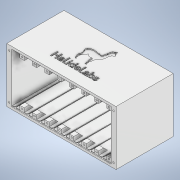
# Autodesk Inventor part: obudowa_główna
Saved by Autodesk Inventor 2020 (Build 240168000, 168)
## iProperties
Created: 2020-04-06
Part Number: obudowa_główna
Material: Tworzywo sztuczne ABS
Document SubType Name: Modeling
Designer: Bartek
Density: 1.06 g/cm^3
Appearance: Gładki — biały
Mass: 835.095 g
Surface Area: 2333.52 cm^2
Volume: 787.826 cm^3
Author: Bartek
Autodesk Inventor part; units mm, degrees
(part 1 of 3)
sketch "Szkic1" plane through (0, 0, 0) normal (0, 0, 1) x (1, 0, 0)
  line L0 (-110, 55) -> (110, 55)
  line L1 (110, 55) -> (110, -55)
  line L2 (110, -55) -> (-110, -55)
  line L3 (-110, -55) -> (-110, 55)
  line L4 (-110, 55) -> (110, -55) construction
  line L5 (110, 55) -> (-110, -55) construction
  point P0 (0, 0)
  dimension "d0" = 220
  dimension "d1" = 110
  constraints: 12 end point, 2 midpoint, 2 parallel, 1 horizontal, 1 perpendicular
  measures "d0" distance of L1.end L2.end
  measures "d1" distance of L0.end L1.end
extrude "Wyciągnięcie proste1" add sketch "Szkic1" along normal blind 115.25
sketch "Szkic2" plane through (0, 0, 115.25) normal (0, 0, 1) x (1, 0, 0)
  line L0 (-110, 55) -> (-110, -55) projected
  line L1 (-95, 50.2) -> (-93.2, 50.2)
  line L2 (-93.2, 50.2) -> (-93.2, 49)
  line L3 (-93.2, 49) -> (-95, 49)
  line L4 (-95, 49) -> (-95, 50.2)
  line L5 (-95, 50.2) -> (-93.2, 49) construction
  line L6 (-93.2, 50.2) -> (-95, 49) construction
  line L7 (110, 55) -> (-110, 55) projected
  line L8 (-70, 49) -> (-70, 50.2)
  line L9 (-68.2, 49) -> (-70, 49)
  line L10 (-68.2, 50.2) -> (-68.2, 49)
  line L11 (-70, 50.2) -> (-68.2, 50.2)
  line L12 (-45, 49) -> (-45, 50.2)
  line L13 (-43.2, 49) -> (-45, 49)
  line L14 (-43.2, 50.2) -> (-43.2, 49)
  line L15 (-45, 50.2) -> (-43.2, 50.2)
  line L16 (-20, 49) -> (-20, 50.2)
  line L17 (-18.2, 49) -> (-20, 49)
  line L18 (-18.2, 50.2) -> (-18.2, 49)
  line L19 (-20, 50.2) -> (-18.2, 50.2)
  line L20 (5, 49) -> (5, 50.2)
  line L21 (6.8, 49) -> (5, 49)
  line L22 (6.8, 50.2) -> (6.8, 49)
  line L23 (5, 50.2) -> (6.8, 50.2)
  line L24 (30, 49) -> (30, 50.2)
  line L25 (31.8, 49) -> (30, 49)
  line L26 (31.8, 50.2) -> (31.8, 49)
  line L27 (30, 50.2) -> (31.8, 50.2)
  line L28 (55, 49) -> (55, 50.2)
  line L29 (56.8, 49) -> (55, 49)
  line L30 (56.8, 50.2) -> (56.8, 49)
  line L31 (55, 50.2) -> (56.8, 50.2)
  line L32 (80, 49) -> (80, 50.2)
  line L33 (81.8, 49) -> (80, 49)
  line L34 (81.8, 50.2) -> (81.8, 49)
  line L35 (80, 50.2) -> (81.8, 50.2)
  line L36 (-110, 0) -> (110, 0)
  line L37 (-95, -50.2) -> (-93.2, -50.2)
  line L38 (-93.2, -50.2) -> (-93.2, -49)
  line L39 (-93.2, -49) -> (-95, -49)
  line L40 (-95, -49) -> (-95, -50.2)
  line L41 (-95, -50.2) -> (-93.2, -49) construction
  line L42 (-93.2, -50.2) -> (-95, -49) construction
  line L43 (-70, -49) -> (-70, -50.2)
  line L44 (-68.2, -49) -> (-70, -49)
  line L45 (-68.2, -50.2) -> (-68.2, -49)
  line L46 (-70, -50.2) -> (-68.2, -50.2)
  line L47 (-45, -49) -> (-45, -50.2)
  line L48 (-43.2, -49) -> (-45, -49)
  line L49 (-43.2, -50.2) -> (-43.2, -49)
  line L50 (-45, -50.2) -> (-43.2, -50.2)
  line L51 (-20, -49) -> (-20, -50.2)
  line L52 (-18.2, -49) -> (-20, -49)
  line L53 (-18.2, -50.2) -> (-18.2, -49)
  line L54 (-20, -50.2) -> (-18.2, -50.2)
  line L55 (5, -49) -> (5, -50.2)
  line L56 (6.8, -49) -> (5, -49)
  line L57 (6.8, -50.2) -> (6.8, -49)
  line L58 (5, -50.2) -> (6.8, -50.2)
  line L59 (30, -49) -> (30, -50.2)
  line L60 (31.8, -49) -> (30, -49)
  line L61 (31.8, -50.2) -> (31.8, -49)
  line L62 (30, -50.2) -> (31.8, -50.2)
  line L63 (55, -49) -> (55, -50.2)
  line L64 (56.8, -49) -> (55, -49)
  line L65 (56.8, -50.2) -> (56.8, -49)
  line L66 (55, -50.2) -> (56.8, -50.2)
  line L67 (80, -49) -> (80, -50.2)
  line L68 (81.8, -49) -> (80, -49)
  line L69 (81.8, -50.2) -> (81.8, -49)
  line L70 (80, -50.2) -> (81.8, -50.2)
  line L71 (-110, -55) -> (110, -55) projected
  point P0 (0, 0)
  point P1 (-94.1, 49.6)
  point P2 (-94.1, -49.6)
  dimension "d7" = 1.8
  dimension "d11" = 15
  dimension "d12" = 4.8
  dimension "d13" = 1.2
  dimension "d17" = 25
  dimension "d56" = 4.8
  dimension "d129" = 1.2
  constraints: 138 end point, 33 symmetric about line, 5 midpoint, 3 horizontal, 2 parallel, 1 collinear, 1 perpendicular, 55 other
  measures "d7" distance between parallel lines of L2 L4
  measures "d11" horizontal distance of L0.start L1.start
  measures "d12" distance between parallel lines of L7 L1
  measures "d13" distance between parallel lines of L1 L3
  measures "d17" distance of L3.end L8.start
  measures "d56" distance from line of L71 L37.start
  measures "d129" distance between parallel lines of L39 L37
extrude "Wyciągnięcie proste2" cut sketch "Szkic2" against normal blind 103.65
sketch "Szkic3" plane through (0, 0, 115.25) normal (0, 0, 1) x (1, 0, 0)
  line L0 (-95, 49) -> (-100, 49)
  line L1 (-100, 49) -> (-100, -49)
  line L2 (-100, -49) -> (100, -49)
  line L3 (100, -49) -> (100, 49)
  line L4 (100, 49) -> (-100, 49)
  line L5 (110, -55) -> (110, 55) projected
  line L6 (-110, 55) -> (-110, -55) projected
  line L7 (110, 55) -> (-110, 55) projected
  point P0 (0, 0)
  dimension "d24" = 5
  dimension "d25" = 98
  dimension "d26" = 200
  dimension "d27" = 98
  dimension "d28" = 90
  dimension "d29" = 10
  dimension "d30" = 10
  dimension "d31" = 6
  dimension "d63" = 6
  constraints: 10 end point, 3 perpendicular, 1 horizontal
  measures "d24" distance of L0.start L0.end
  measures "d25" distance of L0.end L1.end
  measures "d26" distance of L1.end L2.end
  measures "d27" distance of L2.end L3.end
  measures "d28" angle of L3 L2
  measures "d29" distance between parallel lines of L5 L3
  measures "d30" distance between parallel lines of L1 L6
  measures "d31" distance from line of L5.start L2
  measures "d63" distance from line of L7 L0.start
extrude "Wyciągnięcie proste3" cut sketch "Szkic3" against normal blind 106.61
ref_plane "Płaszczyzna konstrukcyjna2" through (0, 0, 115.25) normal (0, 0, 1) x (1, 0, 0)
sketch "Szkic4" plane through (0, 0, 115.25) normal (0, 0, 1) x (1, 0, 0)
  line L0 (-94.1, 52.3714) -> (-94.1, 48.8259)
  line L1 (-93.2, 50.2) -> (-93.2, 49) projected
  line L2 (-95, 49) -> (-95, 50.2) projected
  line L3 (-100, 0) -> (99.7125, 0)
  line L4 (-95, 50.2) -> (-93.2, 50.2) projected
  circle A0 centre (-80.7, 45.2) radius 1.5
  line L5 (-85.1, 49.2) -> (-85.1, 41.2)
  line L6 (-85.1, 41.2) -> (-76.3, 41.2)
  line L7 (-76.3, 41.2) -> (-76.3, 49.2)
  line L8 (-76.3, 49.2) -> (-85.1, 49.2)
  line L9 (-80.6711, 45.15) -> (-80.7289, 45.15)
  line L10 (-80.7289, 45.15) -> (-80.7577, 45.2)
  line L11 (-80.7577, 45.2) -> (-80.7289, 45.25)
  line L12 (-80.7289, 45.25) -> (-80.6711, 45.25)
  line L13 (-80.6711, 45.25) -> (-80.6423, 45.2)
  line L14 (-80.6423, 45.2) -> (-80.6711, 45.15)
  line L15 (-60.1, 49.2) -> (-60.1, 41.2)
  line L16 (-60.1, 41.2) -> (-51.3, 41.2)
  line L17 (-51.3, 49.2) -> (-60.1, 49.2)
  line L18 (-51.3, 41.2) -> (-51.3, 49.2)
  line L19 (-55.6711, 45.25) -> (-55.6423, 45.2)
  line L20 (-55.7289, 45.25) -> (-55.6711, 45.25)
  line L21 (-55.7577, 45.2) -> (-55.7289, 45.25)
  line L22 (-55.7289, 45.15) -> (-55.7577, 45.2)
  line L23 (-55.6711, 45.15) -> (-55.7289, 45.15)
  line L24 (-55.6423, 45.2) -> (-55.6711, 45.15)
  circle A1 centre (-55.7, 45.2) radius 1.5
  line L25 (-35.1, 49.2) -> (-35.1, 41.2)
  line L26 (-35.1, 41.2) -> (-26.3, 41.2)
  line L27 (-26.3, 49.2) -> (-35.1, 49.2)
  line L28 (-26.3, 41.2) -> (-26.3, 49.2)
  line L29 (-30.6711, 45.25) -> (-30.6423, 45.2)
  line L30 (-30.7289, 45.25) -> (-30.6711, 45.25)
  line L31 (-30.7577, 45.2) -> (-30.7289, 45.25)
  line L32 (-30.7289, 45.15) -> (-30.7577, 45.2)
  line L33 (-30.6711, 45.15) -> (-30.7289, 45.15)
  line L34 (-30.6423, 45.2) -> (-30.6711, 45.15)
  circle A2 centre (-30.7, 45.2) radius 1.5
  line L35 (-10.1, 49.2) -> (-10.1, 41.2)
  line L36 (-10.1, 41.2) -> (-1.3, 41.2)
  line L37 (-1.3, 49.2) -> (-10.1, 49.2)
  line L38 (-1.3, 41.2) -> (-1.3, 49.2)
  line L39 (-5.6711, 45.25) -> (-5.6423, 45.2)
  line L40 (-5.7289, 45.25) -> (-5.6711, 45.25)
  line L41 (-5.7577, 45.2) -> (-5.7289, 45.25)
  line L42 (-5.7289, 45.15) -> (-5.7577, 45.2)
  line L43 (-5.6711, 45.15) -> (-5.7289, 45.15)
  line L44 (-5.6423, 45.2) -> (-5.6711, 45.15)
  circle A3 centre (-5.7, 45.2) radius 1.5
  line L45 (14.9, 49.2) -> (14.9, 41.2)
  line L46 (14.9, 41.2) -> (23.7, 41.2)
  line L47 (23.7, 49.2) -> (14.9, 49.2)
  line L48 (23.7, 41.2) -> (23.7, 49.2)
  line L49 (19.3289, 45.25) -> (19.3577, 45.2)
  line L50 (19.2711, 45.25) -> (19.3289, 45.25)
  line L51 (19.2423, 45.2) -> (19.2711, 45.25)
  line L52 (19.2711, 45.15) -> (19.2423, 45.2)
  line L53 (19.3289, 45.15) -> (19.2711, 45.15)
  line L54 (19.3577, 45.2) -> (19.3289, 45.15)
  circle A4 centre (19.3, 45.2) radius 1.5
  line L55 (39.9, 49.2) -> (39.9, 41.2)
  line L56 (39.9, 41.2) -> (48.7, 41.2)
  line L57 (48.7, 49.2) -> (39.9, 49.2)
  line L58 (48.7, 41.2) -> (48.7, 49.2)
  line L59 (44.3289, 45.25) -> (44.3577, 45.2)
  line L60 (44.2711, 45.25) -> (44.3289, 45.25)
  line L61 (44.2423, 45.2) -> (44.2711, 45.25)
  line L62 (44.2711, 45.15) -> (44.2423, 45.2)
  line L63 (44.3289, 45.15) -> (44.2711, 45.15)
  line L64 (44.3577, 45.2) -> (44.3289, 45.15)
  circle A5 centre (44.3, 45.2) radius 1.5
  line L65 (64.9, 49.2) -> (64.9, 41.2)
  line L66 (64.9, 41.2) -> (73.7, 41.2)
  line L67 (73.7, 49.2) -> (64.9, 49.2)
  line L68 (73.7, 41.2) -> (73.7, 49.2)
  line L69 (69.3289, 45.25) -> (69.3577, 45.2)
  line L70 (69.2711, 45.25) -> (69.3289, 45.25)
  line L71 (69.2423, 45.2) -> (69.2711, 45.25)
  line L72 (69.2711, 45.15) -> (69.2423, 45.2)
  line L73 (69.3289, 45.15) -> (69.2711, 45.15)
  line L74 (69.3577, 45.2) -> (69.3289, 45.15)
  circle A6 centre (69.3, 45.2) radius 1.5
  line L75 (89.9, 49.2) -> (89.9, 41.2)
  line L76 (89.9, 41.2) -> (98.7, 41.2)
  line L77 (98.7, 49.2) -> (89.9, 49.2)
  line L78 (98.7, 41.2) -> (98.7, 49.2)
  line L79 (94.3289, 45.25) -> (94.3577, 45.2)
  line L80 (94.2711, 45.25) -> (94.3289, 45.25)
  line L81 (94.2423, 45.2) -> (94.2711, 45.25)
  line L82 (94.2711, 45.15) -> (94.2423, 45.2)
  line L83 (94.3289, 45.15) -> (94.2711, 45.15)
  line L84 (94.3577, 45.2) -> (94.3289, 45.15)
  circle A7 centre (94.3, 45.2) radius 1.5
  line L85 (-94.1, -52.3714) -> (-94.1, -48.8259)
  line L86 (-93.2, -50.2) -> (-93.2, -49)
  line L87 (-95, -49) -> (-95, -50.2)
  line L88 (-95, -50.2) -> (-93.2, -50.2)
  circle A8 centre (-80.7, -45.2) radius 1.5
  line L89 (-85.1, -49.2) -> (-85.1, -41.2)
  line L90 (-85.1, -41.2) -> (-76.3, -41.2)
  line L91 (-76.3, -41.2) -> (-76.3, -49.2)
  line L92 (-76.3, -49.2) -> (-85.1, -49.2)
  line L93 (-80.6711, -45.15) -> (-80.7289, -45.15)
  line L94 (-80.7289, -45.15) -> (-80.7577, -45.2)
  line L95 (-80.7577, -45.2) -> (-80.7289, -45.25)
  line L96 (-80.7289, -45.25) -> (-80.6711, -45.25)
  line L97 (-80.6711, -45.25) -> (-80.6423, -45.2)
  line L98 (-80.6423, -45.2) -> (-80.6711, -45.15)
  line L99 (-60.1, -49.2) -> (-60.1, -41.2)
  line L100 (-60.1, -41.2) -> (-51.3, -41.2)
  line L101 (-51.3, -49.2) -> (-60.1, -49.2)
  line L102 (-51.3, -41.2) -> (-51.3, -49.2)
  line L103 (-55.6711, -45.25) -> (-55.6423, -45.2)
  line L104 (-55.7289, -45.25) -> (-55.6711, -45.25)
  line L105 (-55.7577, -45.2) -> (-55.7289, -45.25)
  line L106 (-55.7289, -45.15) -> (-55.7577, -45.2)
  line L107 (-55.6711, -45.15) -> (-55.7289, -45.15)
  line L108 (-55.6423, -45.2) -> (-55.6711, -45.15)
  circle A9 centre (-55.7, -45.2) radius 1.5
  line L109 (-35.1, -49.2) -> (-35.1, -41.2)
  line L110 (-35.1, -41.2) -> (-26.3, -41.2)
  line L111 (-26.3, -49.2) -> (-35.1, -49.2)
  line L112 (-26.3, -41.2) -> (-26.3, -49.2)
  line L113 (-30.6711, -45.25) -> (-30.6423, -45.2)
  line L114 (-30.7289, -45.25) -> (-30.6711, -45.25)
  line L115 (-30.7577, -45.2) -> (-30.7289, -45.25)
  line L116 (-30.7289, -45.15) -> (-30.7577, -45.2)
  line L117 (-30.6711, -45.15) -> (-30.7289, -45.15)
  line L118 (-30.6423, -45.2) -> (-30.6711, -45.15)
  circle A10 centre (-30.7, -45.2) radius 1.5
  line L119 (-10.1, -49.2) -> (-10.1, -41.2)
  line L120 (-10.1, -41.2) -> (-1.3, -41.2)
  line L121 (-1.3, -49.2) -> (-10.1, -49.2)
  line L122 (-1.3, -41.2) -> (-1.3, -49.2)
  line L123 (-5.6711, -45.25) -> (-5.6423, -45.2)
  line L124 (-5.7289, -45.25) -> (-5.6711, -45.25)
  line L125 (-5.7577, -45.2) -> (-5.7289, -45.25)
  line L126 (-5.7289, -45.15) -> (-5.7577, -45.2)
  line L127 (-5.6711, -45.15) -> (-5.7289, -45.15)
  line L128 (-5.6423, -45.2) -> (-5.6711, -45.15)
  circle A11 centre (-5.7, -45.2) radius 1.5
  line L129 (14.9, -49.2) -> (14.9, -41.2)
  line L130 (14.9, -41.2) -> (23.7, -41.2)
  line L131 (23.7, -49.2) -> (14.9, -49.2)
  line L132 (23.7, -41.2) -> (23.7, -49.2)
  line L133 (19.3289, -45.25) -> (19.3577, -45.2)
  line L134 (19.2711, -45.25) -> (19.3289, -45.25)
  line L135 (19.2423, -45.2) -> (19.2711, -45.25)
  line L136 (19.2711, -45.15) -> (19.2423, -45.2)
  line L137 (19.3289, -45.15) -> (19.2711, -45.15)
  line L138 (19.3577, -45.2) -> (19.3289, -45.15)
  circle A12 centre (19.3, -45.2) radius 1.5
  line L139 (39.9, -49.2) -> (39.9, -41.2)
  line L140 (39.9, -41.2) -> (48.7, -41.2)
  line L141 (48.7, -49.2) -> (39.9, -49.2)
  line L142 (48.7, -41.2) -> (48.7, -49.2)
  line L143 (44.3289, -45.25) -> (44.3577, -45.2)
  line L144 (44.2711, -45.25) -> (44.3289, -45.25)
  line L145 (44.2423, -45.2) -> (44.2711, -45.25)
  line L146 (44.2711, -45.15) -> (44.2423, -45.2)
  line L147 (44.3289, -45.15) -> (44.2711, -45.15)
  line L148 (44.3577, -45.2) -> (44.3289, -45.15)
  circle A13 centre (44.3, -45.2) radius 1.5
  line L149 (64.9, -49.2) -> (64.9, -41.2)
  line L150 (64.9, -41.2) -> (73.7, -41.2)
  line L151 (73.7, -49.2) -> (64.9, -49.2)
  line L152 (73.7, -41.2) -> (73.7, -49.2)
  line L153 (69.3289, -45.25) -> (69.3577, -45.2)
  line L154 (69.2711, -45.25) -> (69.3289, -45.25)
  line L155 (69.2423, -45.2) -> (69.2711, -45.25)
  line L156 (69.2711, -45.15) -> (69.2423, -45.2)
  line L157 (69.3289, -45.15) -> (69.2711, -45.15)
  line L158 (69.3577, -45.2) -> (69.3289, -45.15)
  circle A14 centre (69.3, -45.2) radius 1.5
  line L159 (89.9, -49.2) -> (89.9, -41.2)
  line L160 (89.9, -41.2) -> (98.7, -41.2)
  line L161 (98.7, -49.2) -> (89.9, -49.2)
  line L162 (98.7, -41.2) -> (98.7, -49.2)
  line L163 (94.3289, -45.25) -> (94.3577, -45.2)
  line L164 (94.2711, -45.25) -> (94.3289, -45.25)
  line L165 (94.2423, -45.2) -> (94.2711, -45.25)
  line L166 (94.2711, -45.15) -> (94.2423, -45.2)
  line L167 (94.3289, -45.15) -> (94.2711, -45.15)
  line L168 (94.3577, -45.2) -> (94.3289, -45.15)
  circle A15 centre (94.3, -45.2) radius 1.5
  point P0 (0, 0)
  dimension "d35" = 1.8
  dimension "d36" = 0.9
  dimension "d39" = 3
  dimension "d40" = 5
  dimension "d41" = 13.4
  dimension "d42" = 8
  dimension "d43" = 8.8
  dimension "d44" = 4.4
  dimension "d45" = 14.3
  dimension "d46" = 0.1
  dimension "d49" = 25
  dimension "d64" = 4
  constraints: 332 end point, 95 symmetric about line, 16 centre point, 3 vertical, 2 coincident, 2 horizontal, 2 perpendicular, 1 collinear, 1 parallel, 173 other
  measures "d35" distance between parallel lines of L1 L2
  measures "d36" distance between parallel lines of L0 L2
  measures "d39" diameter of A0
  measures "d40" distance from line of L4 A0.centre
  measures "d41" distance from line of A0.centre L0
  measures "d42" distance of L5.start L5.end
  measures "d43" distance of L5.end L6.end
  measures "d44" distance from line of L5 A0.centre
  measures "d45" distance from line of L2 A0.centre
  measures "d46" vertical distance of L12.end L9.end
  measures "d49" distance of L5.start L15.start
  measures "d64" distance from line of L6 A0.centre
extrude "Wyciągnięcie proste4" add sketch "Szkic4" against normal blind 106.61 contours L8 L7 L6 L5 | L17 L18 L16 L15 | L27 L28 L26 L25 | L37 L38 L36 L35 | L47 L48 L46 L45 | L57 L58 L56 L55 | L67 L68 L66 L65 | L77 L78 L76 L75 | L89 L90 L91 L92 | L99 L100 L102 L101 | L109 L110 L112 L111 | L119 L120 L122 L121 | L129 L130 L132 L131 | L139 L140 L142 L141 | L149 L150 L152 L151 | L159 L160 L162 L161
sketch "Szkic5" plane through (0, 0, 115.25) normal (0, 0, 1) x (1, 0, 0)
  line L0 (100, 49) -> (100, -49) projected
  line L1 (-100, -49) -> (-100, 49) projected
  line L2 (-100, 50.2) -> (100, 50.2)
  line L3 (100, 50.2) -> (100, -50.2)
  line L4 (100, -50.2) -> (-100, -50.2)
  line L5 (-100, -50.2) -> (-100, 50.2)
  line L6 (-100, 50.2) -> (100, -50.2) construction
  line L7 (100, 50.2) -> (-100, -50.2) construction
  point P0 (0, 0)
  point P1 (100, -49)
  point P2 (-100, 49)
  point P3 (-100, -49)
  dimension "d57" = 200
  dimension "d58" = 98
  dimension "d59" = 200
  dimension "d60" = 100.4
  constraints: 12 end point, 2 midpoint, 2 parallel, 1 horizontal, 1 perpendicular
  measures "d57" distance between parallel lines of L0 L1
  measures "d58" distance of L1.end L1.start
  measures "d59" distance between parallel lines of L3 L5
  measures "d60" distance between parallel lines of L2 L4
extrude "Wyciągnięcie proste5" cut sketch "Szkic5" against normal blind 1.6
ref_plane "Płaszczyzna konstrukcyjna5" through (-51.3, -49, 10) normal (0, 1, 0) x (1, 0, 0)
sketch "Szkic7" plane through (-51.3, -49, 10) normal (0, 1, 0) x (1, 0, 0)
  line L0 (-44.5014, -102.9088) -> (-43.7341, -100.0451)
  line L1 (-44.8189, -104.0803) -> (-39.2569, -104.0803) construction
  line L2 (-42.8, -98.9304) -> (-42.8, -103.8241)
  line L3 (-41.9, -103.65) -> (-41.9, -1.6) projected
  arc A0 (-43.7341, -100.0451) -> (-43.7, -99.7863) centre (-44.7, -99.7863) ccw
  line L4 (-43.7, -103.65) -> (-43.7, -99.7863)
  line L5 (-43.7, -103.65) -> (-43.7, -1.6) projected
  arc A1 (-45.4673, -103.65) -> (-44.5014, -102.9088) centre (-45.4673, -102.65) ccw
  line L6 (-43.7, -103.65) -> (-45.4673, -103.65)
  line L7 (-41.0986, -102.9088) -> (-41.8659, -100.0451)
  arc A2 (-41.9, -99.7863) -> (-41.8659, -100.0451) centre (-40.9, -99.7863) ccw
  line L8 (-41.9, -103.65) -> (-41.9, -99.7863)
  arc A3 (-41.0986, -102.9088) -> (-40.1327, -103.65) centre (-40.1327, -102.65) ccw
  line L9 (-41.9, -103.65) -> (-40.1327, -103.65)
  line L10 (-19.5014, -102.9088) -> (-18.7341, -100.0451)
  arc A4 (-20.4673, -103.65) -> (-19.5014, -102.9088) centre (-20.4673, -102.65) ccw
  line L11 (-18.7, -103.65) -> (-18.7, -99.7863)
  arc A5 (-18.7341, -100.0451) -> (-18.7, -99.7863) centre (-19.7, -99.7863) ccw
  line L12 (-18.7, -103.65) -> (-20.4673, -103.65)
  arc A6 (-16.9, -99.7863) -> (-16.8659, -100.0451) centre (-15.9, -99.7863) ccw
  line L13 (-16.9, -103.65) -> (-16.9, -99.7863)
  line L14 (-16.0986, -102.9088) -> (-16.8659, -100.0451)
  arc A7 (-16.0986, -102.9088) -> (-15.1327, -103.65) centre (-15.1327, -102.65) ccw
  line L15 (-16.9, -103.65) -> (-15.1327, -103.65)
  line L16 (5.4986, -102.9088) -> (6.2659, -100.0451)
  arc A8 (4.5327, -103.65) -> (5.4986, -102.9088) centre (4.5327, -102.65) ccw
  line L17 (6.3, -103.65) -> (6.3, -99.7863)
  arc A9 (6.2659, -100.0451) -> (6.3, -99.7863) centre (5.3, -99.7863) ccw
  line L18 (6.3, -103.65) -> (4.5327, -103.65)
  arc A10 (8.1, -99.7863) -> (8.1341, -100.0451) centre (9.1, -99.7863) ccw
  line L19 (8.1, -103.65) -> (8.1, -99.7863)
  line L20 (8.9014, -102.9088) -> (8.1341, -100.0451)
  arc A11 (8.9014, -102.9088) -> (9.8673, -103.65) centre (9.8673, -102.65) ccw
  line L21 (8.1, -103.65) -> (9.8673, -103.65)
  line L22 (30.4986, -102.9088) -> (31.2659, -100.0451)
  arc A12 (29.5327, -103.65) -> (30.4986, -102.9088) centre (29.5327, -102.65) ccw
  line L23 (31.3, -103.65) -> (31.3, -99.7863)
  arc A13 (31.2659, -100.0451) -> (31.3, -99.7863) centre (30.3, -99.7863) ccw
  line L24 (31.3, -103.65) -> (29.5327, -103.65)
  arc A14 (33.1, -99.7863) -> (33.1341, -100.0451) centre (34.1, -99.7863) ccw
  line L25 (33.1, -103.65) -> (33.1, -99.7863)
  line L26 (33.9014, -102.9088) -> (33.1341, -100.0451)
  arc A15 (33.9014, -102.9088) -> (34.8673, -103.65) centre (34.8673, -102.65) ccw
  line L27 (33.1, -103.65) -> (34.8673, -103.65)
  line L28 (55.4986, -102.9088) -> (56.2659, -100.0451)
  arc A16 (54.5327, -103.65) -> (55.4986, -102.9088) centre (54.5327, -102.65) ccw
  line L29 (56.3, -103.65) -> (56.3, -99.7863)
  arc A17 (56.2659, -100.0451) -> (56.3, -99.7863) centre (55.3, -99.7863) ccw
  line L30 (56.3, -103.65) -> (54.5327, -103.65)
  arc A18 (58.1, -99.7863) -> (58.1341, -100.0451) centre (59.1, -99.7863) ccw
  line L31 (58.1, -103.65) -> (58.1, -99.7863)
  line L32 (58.9014, -102.9088) -> (58.1341, -100.0451)
  arc A19 (58.9014, -102.9088) -> (59.8673, -103.65) centre (59.8673, -102.65) ccw
  line L33 (58.1, -103.65) -> (59.8673, -103.65)
  line L34 (80.4986, -102.9088) -> (81.2659, -100.0451)
  arc A20 (79.5327, -103.65) -> (80.4986, -102.9088) centre (79.5327, -102.65) ccw
  line L35 (81.3, -103.65) -> (81.3, -99.7863)
  arc A21 (81.2659, -100.0451) -> (81.3, -99.7863) centre (80.3, -99.7863) ccw
  line L36 (81.3, -103.65) -> (79.5327, -103.65)
  arc A22 (83.1, -99.7863) -> (83.1341, -100.0451) centre (84.1, -99.7863) ccw
  line L37 (83.1, -103.65) -> (83.1, -99.7863)
  line L38 (83.9014, -102.9088) -> (83.1341, -100.0451)
  arc A23 (83.9014, -102.9088) -> (84.8673, -103.65) centre (84.8673, -102.65) ccw
  line L39 (83.1, -103.65) -> (84.8673, -103.65)
  line L40 (105.4986, -102.9088) -> (106.2659, -100.0451)
  arc A24 (104.5327, -103.65) -> (105.4986, -102.9088) centre (104.5327, -102.65) ccw
  line L41 (106.3, -103.65) -> (106.3, -99.7863)
  arc A25 (106.2659, -100.0451) -> (106.3, -99.7863) centre (105.3, -99.7863) ccw
  line L42 (106.3, -103.65) -> (104.5327, -103.65)
  arc A26 (108.1, -99.7863) -> (108.1341, -100.0451) centre (109.1, -99.7863) ccw
  line L43 (108.1, -103.65) -> (108.1, -99.7863)
  line L44 (108.9014, -102.9088) -> (108.1341, -100.0451)
  arc A27 (108.9014, -102.9088) -> (109.8673, -103.65) centre (109.8673, -102.65) ccw
  line L45 (108.1, -103.65) -> (109.8673, -103.65)
  line L46 (130.4986, -102.9088) -> (131.2659, -100.0451)
  arc A28 (129.5327, -103.65) -> (130.4986, -102.9088) centre (129.5327, -102.65) ccw
  line L47 (131.3, -103.65) -> (131.3, -99.7863)
  arc A29 (131.2659, -100.0451) -> (131.3, -99.7863) centre (130.3, -99.7863) ccw
  line L48 (131.3, -103.65) -> (129.5327, -103.65)
  arc A30 (133.1, -99.7863) -> (133.1341, -100.0451) centre (134.1, -99.7863) ccw
  line L49 (133.1, -103.65) -> (133.1, -99.7863)
  line L50 (133.9014, -102.9088) -> (133.1341, -100.0451)
  arc A31 (133.9014, -102.9088) -> (134.8673, -103.65) centre (134.8673, -102.65) ccw
  line L51 (133.1, -103.65) -> (134.8673, -103.65)
  point P0 (51.3, 10)
  point P1 (-40.7811, -104.0803)
  point P2 (-19.8189, -104.0803)
  point P3 (-15.7811, -104.0803)
  point P4 (5.1811, -104.0803)
  point P5 (9.2189, -104.0803)
  point P6 (30.1811, -104.0803)
  point P7 (34.2189, -104.0803)
  point P8 (55.1811, -104.0803)
  point P9 (59.2189, -104.0803)
  point P10 (80.1811, -104.0803)
  point P11 (84.2189, -104.0803)
  point P12 (105.1811, -104.0803)
  point P13 (109.2189, -104.0803)
  point P14 (130.1811, -104.0803)
  point P15 (134.2189, -104.0803)
  point P16 (-41.9, -99.7863)
  dimension "d80" = 1
  dimension "d81" = 1
  dimension "d84" = 25
  dimension "d89" = 1.7673
  dimension "d90" = 3.8637
  dimension "d91" = 1.8
  dimension "d92" = 0.9
  constraints: 100 end point, 64 point on circle, 32 centre point, 7 symmetric about line, 2 horizontal, 2 tangent, 1 collinear, 1 vertical, 183 other
  measures "d80" radius of A0
  measures "d81" radius of A1
  measures "d84" distance of L0.start L10.start
  measures "d89" distance of L4.start L6.end
  measures "d90" distance from line of L6 L4.end
  measures "d91" distance from line of L8 L4.start
  measures "d92" distance from line of L2 L4.start
extrude "Wyciągnięcie proste6" cut sketch "Szkic7" against normal up to surface (1.2 mm away)
ref_plane "Płaszczyzna konstrukcyjna7" through (-100, 49, 8.64) normal (0, -1, 0) x (1, 0, 0)
sketch "Szkic8" plane through (-100, 49, 8.64) normal (0, -1, 0) x (1, 0, 0)
  line L0 (0, 105.01) -> (5, 105.01) projected
  line L1 (5, 105.01) -> (5, 2.96) projected
  line L2 (5, 2.96) -> (6.8, 2.96) projected
  line L3 (6.8, 2.96) -> (6.8, 105.01) projected
  line L4 (6.8, 105.01) -> (14.9, 105.01) projected
  line L5 (14.9, 105.01) -> (23.7, 105.01) projected
  line L6 (23.7, 105.01) -> (23.7, 0) projected
  line L7 (39.9, 0) -> (39.9, 105.01) projected
  line L8 (31.8, 105.01) -> (39.9, 105.01) projected
  line L9 (31.8, 2.96) -> (31.8, 105.01) projected
  line L10 (30, 2.96) -> (31.8, 2.96) projected
  line L11 (30, 105.01) -> (30, 2.96) projected
  line L12 (23.7, 105.01) -> (30, 105.01) projected
  line L13 (0, 105.01) -> (0, 0) projected
  line L14 (0, 106.61) -> (0, 105.01) projected
  line L15 (-10, 106.61) -> (0, 106.61) projected
  line L16 (-10, -8.64) -> (-10, 106.61) projected
  line L17 (210, -8.64) -> (-10, -8.64) projected
  line L18 (210, 106.61) -> (210, -8.64) projected
  line L19 (200, 106.61) -> (210, 106.61) projected
  line L20 (200, 105.01) -> (200, 106.61) projected
  line L21 (198.7, 105.01) -> (200, 105.01) projected
  line L22 (198.7, 105.01) -> (198.7, 0) projected
  line L23 (200, 0) -> (200, 105.01) projected
  line L24 (14.9, 0) -> (14.9, 105.01) projected
  line L25 (0, 0) -> (14.9, 0) projected
  line L26 (39.9, 105.01) -> (48.7, 105.01) projected
  line L27 (48.7, 105.01) -> (48.7, 0) projected
  line L28 (64.9, 0) -> (64.9, 105.01) projected
  line L29 (56.8, 105.01) -> (64.9, 105.01) projected
  line L30 (56.8, 2.96) -> (56.8, 105.01) projected
  line L31 (55, 2.96) -> (56.8, 2.96) projected
  line L32 (55, 105.01) -> (55, 2.96) projected
  line L33 (48.7, 105.01) -> (55, 105.01) projected
  line L34 (189.9, 105.01) -> (198.7, 105.01) projected
  line L35 (189.9, 0) -> (189.9, 105.01) projected
  line L36 (173.7, 105.01) -> (173.7, 0) projected
  line L37 (164.9, 105.01) -> (173.7, 105.01) projected
  line L38 (164.9, 0) -> (164.9, 105.01) projected
  line L39 (148.7, 105.01) -> (148.7, 0) projected
  line L40 (139.9, 105.01) -> (148.7, 105.01) projected
  line L41 (139.9, 0) -> (139.9, 105.01) projected
  line L42 (123.7, 105.01) -> (123.7, 0) projected
  line L43 (123.7, 105.01) -> (130, 105.01) projected
  line L44 (130, 105.01) -> (130, 2.96) projected
  line L45 (130, 2.96) -> (131.8, 2.96) projected
  line L46 (131.8, 2.96) -> (131.8, 105.01) projected
  line L47 (131.8, 105.01) -> (139.9, 105.01) projected
  line L48 (64.9, 105.01) -> (73.7, 105.01) projected
  line L49 (73.7, 105.01) -> (73.7, 0) projected
  line L50 (89.9, 0) -> (89.9, 105.01) projected
  line L51 (81.8, 105.01) -> (89.9, 105.01) projected
  line L52 (81.8, 2.96) -> (81.8, 105.01) projected
  line L53 (80, 2.96) -> (81.8, 2.96) projected
  line L54 (80, 105.01) -> (80, 2.96) projected
  line L55 (73.7, 105.01) -> (80, 105.01) projected
  line L56 (181.8, 105.01) -> (189.9, 105.01) projected
  line L57 (181.8, 2.96) -> (181.8, 105.01) projected
  line L58 (180, 2.96) -> (181.8, 2.96) projected
  line L59 (180, 105.01) -> (180, 2.96) projected
  line L60 (173.7, 105.01) -> (180, 105.01) projected
  line L61 (156.8, 105.01) -> (164.9, 105.01) projected
  line L62 (156.8, 2.96) -> (156.8, 105.01) projected
  line L63 (155, 2.96) -> (156.8, 2.96) projected
  line L64 (155, 105.01) -> (155, 2.96) projected
  line L65 (148.7, 105.01) -> (155, 105.01) projected
  line L66 (114.9, 105.01) -> (123.7, 105.01) projected
  line L67 (114.9, 0) -> (114.9, 105.01) projected
  line L68 (98.7, 105.01) -> (98.7, 0) projected
  line L69 (98.7, 105.01) -> (105, 105.01) projected
  line L70 (105, 105.01) -> (105, 2.96) projected
  line L71 (105, 2.96) -> (106.8, 2.96) projected
  line L72 (106.8, 2.96) -> (106.8, 105.01) projected
  line L73 (106.8, 105.01) -> (114.9, 105.01) projected
  line L74 (89.9, 105.01) -> (98.7, 105.01) projected
  line L75 (0, 105.01) -> (5, 105.01) projected
  line L76 (5, 105.01) -> (5, 2.96) projected
  line L77 (5, 2.96) -> (6.8, 2.96) projected
  line L78 (0, 105.01) -> (0, 0) projected
  line L79 (0, 106.61) -> (0, 105.01) projected
  line L80 (200, 0) -> (200, 105.01) projected
  line L81 (0, 0) -> (14.9, 0) projected
  line L82 (0, 105.01) -> (5, 105.01) projected
  line L83 (5, 105.01) -> (5, 2.96) projected
  line L84 (5, 2.96) -> (6.8, 2.96) projected
  line L85 (0, 105.01) -> (0, 0) projected
  line L86 (0, 106.61) -> (0, 105.01) projected
  line L87 (200, 0) -> (200, 105.01) projected
  line L88 (0, 0) -> (14.9, 0) projected
  line L89 (0, 105.01) -> (5, 105.01) projected
  line L90 (5, 105.01) -> (5, 2.96) projected
  line L91 (5, 2.96) -> (6.8, 2.96) projected
  line L92 (0, 105.01) -> (0, 0) projected
  line L93 (0, 106.61) -> (0, 105.01) projected
  line L94 (200, 0) -> (200, 105.01) projected
  line L95 (0, 0) -> (14.9, 0) projected
  line L96 (0, 105.01) -> (5, 105.01) projected
  line L97 (5, 105.01) -> (5, 2.96) projected
  line L98 (5, 2.96) -> (6.8, 2.96) projected
  line L99 (0, 105.01) -> (0, 0) projected
  line L100 (0, 106.61) -> (0, 105.01) projected
  line L101 (200, 0) -> (200, 105.01) projected
  line L102 (0, 0) -> (14.9, 0) projected
  line L103 (0, 105.01) -> (5, 105.01) projected
  line L104 (5, 105.01) -> (5, 2.96) projected
  line L105 (5, 2.96) -> (6.8, 2.96) projected
  line L106 (0, 105.01) -> (0, 0) projected
  line L107 (0, 106.61) -> (0, 105.01) projected
  line L108 (200, 0) -> (200, 105.01) projected
  line L109 (0, 0) -> (14.9, 0) projected
  line L110 (4.1986, 104.2688) -> (4.9659, 101.4051) projected
  arc A0 (5, 101.1463) -> (4.9659, 101.4051) centre (4, 101.1463) ccw projected
  arc A1 (4.1986, 104.2688) -> (3.2327, 105.01) centre (3.2327, 104.01) ccw projected
  line L111 (5, 105.01) -> (5, 2.96) projected
  line L112 (5, 105.01) -> (3.2327, 105.01)
  line L113 (0, 105.01) -> (5, 105.01) projected
  line L114 (5, 105.01) -> (5, 101.1463)
  line L115 (5.9, 104.5443) -> (5.9, 100.4671)
  line L116 (7.6014, 104.2688) -> (6.8341, 101.4051)
  arc A2 (6.8341, 101.4051) -> (6.8, 101.1463) centre (7.8, 101.1463) ccw
  arc A3 (8.5673, 105.01) -> (7.6014, 104.2688) centre (8.5673, 104.01) ccw
  line L117 (6.8, 105.01) -> (8.5673, 105.01)
  line L118 (6.8, 105.01) -> (6.8, 101.1463)
  line L119 (4.1986, 104.2688) -> (4.9659, 101.4051)
  arc A4 (4.1986, 104.2688) -> (3.2327, 105.01) centre (3.2327, 104.01) ccw
  arc A5 (5, 101.1463) -> (4.9659, 101.4051) centre (4, 101.1463) ccw
  line L120 (30, 105.01) -> (30, 101.1463)
  arc A6 (30, 101.1463) -> (29.9659, 101.4051) centre (29, 101.1463) ccw
  line L121 (30, 105.01) -> (28.2327, 105.01)
  arc A7 (29.1986, 104.2688) -> (28.2327, 105.01) centre (28.2327, 104.01) ccw
  line L122 (29.1986, 104.2688) -> (29.9659, 101.4051)
  arc A8 (33.5673, 105.01) -> (32.6014, 104.2688) centre (33.5673, 104.01) ccw
  line L123 (32.6014, 104.2688) -> (31.8341, 101.4051)
  line L124 (31.8, 105.01) -> (31.8, 101.1463)
  arc A9 (31.8341, 101.4051) -> (31.8, 101.1463) centre (32.8, 101.1463) ccw
  line L125 (31.8, 105.01) -> (33.5673, 105.01)
  line L126 (55, 105.01) -> (55, 101.1463)
  arc A10 (55, 101.1463) -> (54.9659, 101.4051) centre (54, 101.1463) ccw
  line L127 (55, 105.01) -> (53.2327, 105.01)
  arc A11 (54.1986, 104.2688) -> (53.2327, 105.01) centre (53.2327, 104.01) ccw
  line L128 (54.1986, 104.2688) -> (54.9659, 101.4051)
  arc A12 (58.5673, 105.01) -> (57.6014, 104.2688) centre (58.5673, 104.01) ccw
  line L129 (57.6014, 104.2688) -> (56.8341, 101.4051)
  line L130 (56.8, 105.01) -> (56.8, 101.1463)
  arc A13 (56.8341, 101.4051) -> (56.8, 101.1463) centre (57.8, 101.1463) ccw
  line L131 (56.8, 105.01) -> (58.5673, 105.01)
  line L132 (80, 105.01) -> (80, 101.1463)
  arc A14 (80, 101.1463) -> (79.9659, 101.4051) centre (79, 101.1463) ccw
  line L133 (80, 105.01) -> (78.2327, 105.01)
  arc A15 (79.1986, 104.2688) -> (78.2327, 105.01) centre (78.2327, 104.01) ccw
  line L134 (79.1986, 104.2688) -> (79.9659, 101.4051)
  arc A16 (83.5673, 105.01) -> (82.6014, 104.2688) centre (83.5673, 104.01) ccw
  line L135 (82.6014, 104.2688) -> (81.8341, 101.4051)
  line L136 (81.8, 105.01) -> (81.8, 101.1463)
  arc A17 (81.8341, 101.4051) -> (81.8, 101.1463) centre (82.8, 101.1463) ccw
  line L137 (81.8, 105.01) -> (83.5673, 105.01)
  line L138 (105, 105.01) -> (105, 101.1463)
  arc A18 (105, 101.1463) -> (104.9659, 101.4051) centre (104, 101.1463) ccw
  line L139 (105, 105.01) -> (103.2327, 105.01)
  arc A19 (104.1986, 104.2688) -> (103.2327, 105.01) centre (103.2327, 104.01) ccw
  line L140 (104.1986, 104.2688) -> (104.9659, 101.4051)
  arc A20 (108.5673, 105.01) -> (107.6014, 104.2688) centre (108.5673, 104.01) ccw
  line L141 (107.6014, 104.2688) -> (106.8341, 101.4051)
  line L142 (106.8, 105.01) -> (106.8, 101.1463)
  arc A21 (106.8341, 101.4051) -> (106.8, 101.1463) centre (107.8, 101.1463) ccw
  line L143 (106.8, 105.01) -> (108.5673, 105.01)
  line L144 (130, 105.01) -> (130, 101.1463)
  arc A22 (130, 101.1463) -> (129.9659, 101.4051) centre (129, 101.1463) ccw
  line L145 (130, 105.01) -> (128.2327, 105.01)
  arc A23 (129.1986, 104.2688) -> (128.2327, 105.01) centre (128.2327, 104.01) ccw
  line L146 (129.1986, 104.2688) -> (129.9659, 101.4051)
  arc A24 (133.5673, 105.01) -> (132.6014, 104.2688) centre (133.5673, 104.01) ccw
  line L147 (132.6014, 104.2688) -> (131.8341, 101.4051)
  line L148 (131.8, 105.01) -> (131.8, 101.1463)
  arc A25 (131.8341, 101.4051) -> (131.8, 101.1463) centre (132.8, 101.1463) ccw
  line L149 (131.8, 105.01) -> (133.5673, 105.01)
  line L150 (155, 105.01) -> (155, 101.1463)
  arc A26 (155, 101.1463) -> (154.9659, 101.4051) centre (154, 101.1463) ccw
  line L151 (155, 105.01) -> (153.2327, 105.01)
  arc A27 (154.1986, 104.2688) -> (153.2327, 105.01) centre (153.2327, 104.01) ccw
  line L152 (154.1986, 104.2688) -> (154.9659, 101.4051)
  arc A28 (158.5673, 105.01) -> (157.6014, 104.2688) centre (158.5673, 104.01) ccw
  line L153 (157.6014, 104.2688) -> (156.8341, 101.4051)
  line L154 (156.8, 105.01) -> (156.8, 101.1463)
  arc A29 (156.8341, 101.4051) -> (156.8, 101.1463) centre (157.8, 101.1463) ccw
  line L155 (156.8, 105.01) -> (158.5673, 105.01)
  line L156 (180, 105.01) -> (180, 101.1463)
  arc A30 (180, 101.1463) -> (179.9659, 101.4051) centre (179, 101.1463) ccw
  line L157 (180, 105.01) -> (178.2327, 105.01)
  arc A31 (179.1986, 104.2688) -> (178.2327, 105.01) centre (178.2327, 104.01) ccw
  line L158 (179.1986, 104.2688) -> (179.9659, 101.4051)
  arc A32 (183.5673, 105.01) -> (182.6014, 104.2688) centre (183.5673, 104.01) ccw
  line L159 (182.6014, 104.2688) -> (181.8341, 101.4051)
  line L160 (181.8, 105.01) -> (181.8, 101.1463)
  arc A33 (181.8341, 101.4051) -> (181.8, 101.1463) centre (182.8, 101.1463) ccw
  line L161 (181.8, 105.01) -> (183.5673, 105.01)
  line L162 (200, 106.61) -> (210, 106.61) projected
  line L163 (210, 106.61) -> (210, -8.64) projected
  line L164 (210, -8.64) -> (-10, -8.64) projected
  line L165 (-10, -8.64) -> (-10, 106.61) projected
  line L166 (-10, 106.61) -> (0, 106.61) projected
  line L167 (200, 105.01) -> (200, 106.61) projected
  line L168 (6.8, 2.96) -> (6.8, 105.01) projected
  line L169 (6.8, 105.01) -> (14.9, 105.01) projected
  line L170 (14.9, 0) -> (14.9, 105.01) projected
  line L171 (23.7, 105.01) -> (23.7, 0) projected
  line L172 (23.7, 105.01) -> (30, 105.01) projected
  line L173 (30, 105.01) -> (30, 2.96) projected
  line L174 (30, 2.96) -> (31.8, 2.96) projected
  line L175 (31.8, 2.96) -> (31.8, 105.01) projected
  line L176 (31.8, 105.01) -> (39.9, 105.01) projected
  line L177 (39.9, 0) -> (39.9, 105.01) projected
  line L178 (48.7, 105.01) -> (48.7, 0) projected
  line L179 (48.7, 105.01) -> (55, 105.01) projected
  line L180 (55, 105.01) -> (55, 2.96) projected
  line L181 (55, 2.96) -> (56.8, 2.96) projected
  line L182 (56.8, 2.96) -> (56.8, 105.01) projected
  line L183 (56.8, 105.01) -> (64.9, 105.01) projected
  line L184 (64.9, 0) -> (64.9, 105.01) projected
  line L185 (73.7, 105.01) -> (73.7, 0) projected
  line L186 (73.7, 105.01) -> (80, 105.01) projected
  line L187 (80, 105.01) -> (80, 2.96) projected
  line L188 (80, 2.96) -> (81.8, 2.96) projected
  line L189 (81.8, 2.96) -> (81.8, 105.01) projected
  line L190 (81.8, 105.01) -> (89.9, 105.01) projected
  line L191 (89.9, 0) -> (89.9, 105.01) projected
  line L192 (98.7, 105.01) -> (98.7, 0) projected
  line L193 (89.9, 105.01) -> (98.7, 105.01) projected
  line L194 (198.7, 105.01) -> (200, 105.01) projected
  line L195 (198.7, 105.01) -> (198.7, 0) projected
  line L196 (189.9, 0) -> (189.9, 105.01) projected
  line L197 (181.8, 105.01) -> (189.9, 105.01) projected
  line L198 (181.8, 2.96) -> (181.8, 105.01) projected
  line L199 (180, 2.96) -> (181.8, 2.96) projected
  line L200 (180, 105.01) -> (180, 2.96) projected
  line L201 (173.7, 105.01) -> (180, 105.01) projected
  line L202 (173.7, 105.01) -> (173.7, 0) projected
  line L203 (164.9, 0) -> (164.9, 105.01) projected
  line L204 (156.8, 105.01) -> (164.9, 105.01) projected
  line L205 (156.8, 2.96) -> (156.8, 105.01) projected
  line L206 (155, 2.96) -> (156.8, 2.96) projected
  line L207 (155, 105.01) -> (155, 2.96) projected
  line L208 (148.7, 105.01) -> (155, 105.01) projected
  line L209 (148.7, 105.01) -> (148.7, 0) projected
  line L210 (139.9, 0) -> (139.9, 105.01) projected
  line L211 (131.8, 105.01) -> (139.9, 105.01) projected
  line L212 (131.8, 2.96) -> (131.8, 105.01) projected
  line L213 (130, 2.96) -> (131.8, 2.96) projected
  line L214 (130, 105.01) -> (130, 2.96) projected
  line L215 (123.7, 105.01) -> (130, 105.01) projected
  line L216 (123.7, 105.01) -> (123.7, 0) projected
  line L217 (114.9, 0) -> (114.9, 105.01) projected
  line L218 (106.8, 105.01) -> (114.9, 105.01) projected
  line L219 (106.8, 2.96) -> (106.8, 105.01) projected
  line L220 (105, 2.96) -> (106.8, 2.96) projected
  line L221 (105, 105.01) -> (105, 2.96) projected
  line L222 (98.7, 105.01) -> (105, 105.01) projected
  line L223 (14.9, 105.01) -> (23.7, 105.01) projected
  line L224 (39.9, 105.01) -> (48.7, 105.01) projected
  line L225 (64.9, 105.01) -> (73.7, 105.01) projected
  line L226 (189.9, 105.01) -> (198.7, 105.01) projected
  line L227 (164.9, 105.01) -> (173.7, 105.01) projected
  line L228 (139.9, 105.01) -> (148.7, 105.01) projected
  line L229 (114.9, 105.01) -> (123.7, 105.01) projected
  line L230 (14.9, 0) -> (14.9, 105.01) projected
  line L231 (23.7, 105.01) -> (23.7, 0) projected
  line L232 (39.9, 0) -> (39.9, 105.01) projected
  line L233 (48.7, 105.01) -> (48.7, 0) projected
  line L234 (64.9, 0) -> (64.9, 105.01) projected
  line L235 (73.7, 105.01) -> (73.7, 0) projected
  line L236 (89.9, 0) -> (89.9, 105.01) projected
  line L237 (98.7, 105.01) -> (98.7, 0) projected
  line L238 (198.7, 105.01) -> (198.7, 0) projected
  line L239 (189.9, 0) -> (189.9, 105.01) projected
  line L240 (173.7, 105.01) -> (173.7, 0) projected
  line L241 (164.9, 0) -> (164.9, 105.01) projected
  line L242 (148.7, 105.01) -> (148.7, 0) projected
  line L243 (139.9, 0) -> (139.9, 105.01) projected
  line L244 (123.7, 105.01) -> (123.7, 0) projected
  line L245 (114.9, 0) -> (114.9, 105.01) projected
  line L246 (14.9, 0) -> (14.9, 105.01) projected
  line L247 (23.7, 105.01) -> (23.7, 0) projected
  line L248 (39.9, 0) -> (39.9, 105.01) projected
  line L249 (48.7, 105.01) -> (48.7, 0) projected
  line L250 (64.9, 0) -> (64.9, 105.01) projected
  line L251 (73.7, 105.01) -> (73.7, 0) projected
  line L252 (89.9, 0) -> (89.9, 105.01) projected
  line L253 (98.7, 105.01) -> (98.7, 0) projected
  line L254 (198.7, 105.01) -> (198.7, 0) projected
  line L255 (189.9, 0) -> (189.9, 105.01) projected
  line L256 (173.7, 105.01) -> (173.7, 0) projected
  line L257 (164.9, 0) -> (164.9, 105.01) projected
  line L258 (148.7, 105.01) -> (148.7, 0) projected
  line L259 (139.9, 0) -> (139.9, 105.01) projected
  line L260 (123.7, 105.01) -> (123.7, 0) projected
  line L261 (114.9, 0) -> (114.9, 105.01) projected
  line L262 (14.9, 0) -> (14.9, 105.01) projected
  line L263 (23.7, 105.01) -> (23.7, 0) projected
  line L264 (39.9, 0) -> (39.9, 105.01) projected
  line L265 (48.7, 105.01) -> (48.7, 0) projected
  line L266 (64.9, 0) -> (64.9, 105.01) projected
  line L267 (73.7, 105.01) -> (73.7, 0) projected
  line L268 (89.9, 0) -> (89.9, 105.01) projected
  line L269 (98.7, 105.01) -> (98.7, 0) projected
  line L270 (198.7, 105.01) -> (198.7, 0) projected
  line L271 (189.9, 0) -> (189.9, 105.01) projected
  line L272 (173.7, 105.01) -> (173.7, 0) projected
  line L273 (164.9, 0) -> (164.9, 105.01) projected
  line L274 (148.7, 105.01) -> (148.7, 0) projected
  line L275 (139.9, 0) -> (139.9, 105.01) projected
  line L276 (123.7, 105.01) -> (123.7, 0) projected
  line L277 (114.9, 0) -> (114.9, 105.01) projected
  line L278 (14.9, 0) -> (14.9, 105.01) projected
  line L279 (23.7, 105.01) -> (23.7, 0) projected
  line L280 (39.9, 0) -> (39.9, 105.01) projected
  line L281 (48.7, 105.01) -> (48.7, 0) projected
  line L282 (64.9, 0) -> (64.9, 105.01) projected
  line L283 (73.7, 105.01) -> (73.7, 0) projected
  line L284 (89.9, 0) -> (89.9, 105.01) projected
  line L285 (98.7, 105.01) -> (98.7, 0) projected
  line L286 (198.7, 105.01) -> (198.7, 0) projected
  line L287 (189.9, 0) -> (189.9, 105.01) projected
  line L288 (173.7, 105.01) -> (173.7, 0) projected
  line L289 (164.9, 0) -> (164.9, 105.01) projected
  line L290 (148.7, 105.01) -> (148.7, 0) projected
  line L291 (139.9, 0) -> (139.9, 105.01) projected
  line L292 (123.7, 105.01) -> (123.7, 0) projected
  line L293 (114.9, 0) -> (114.9, 105.01) projected
  line L294 (200, 106.61) -> (210, 106.61) projected
  line L295 (210, 106.61) -> (210, -8.64) projected
  line L296 (210, -8.64) -> (-10, -8.64) projected
  line L297 (-10, -8.64) -> (-10, 106.61) projected
  line L298 (-10, 106.61) -> (0, 106.61) projected
  line L299 (200, 105.01) -> (200, 106.61) projected
  line L300 (6.8, 2.96) -> (6.8, 105.01) projected
  line L301 (6.8, 105.01) -> (14.9, 105.01) projected
  line L302 (23.7, 105.01) -> (30, 105.01) projected
  line L303 (30, 105.01) -> (30, 2.96) projected
  line L304 (30, 2.96) -> (31.8, 2.96) projected
  line L305 (31.8, 2.96) -> (31.8, 105.01) projected
  line L306 (31.8, 105.01) -> (39.9, 105.01) projected
  line L307 (48.7, 105.01) -> (55, 105.01) projected
  line L308 (55, 105.01) -> (55, 2.96) projected
  line L309 (55, 2.96) -> (56.8, 2.96) projected
  line L310 (56.8, 2.96) -> (56.8, 105.01) projected
  line L311 (56.8, 105.01) -> (64.9, 105.01) projected
  line L312 (73.7, 105.01) -> (80, 105.01) projected
  line L313 (80, 105.01) -> (80, 2.96) projected
  line L314 (80, 2.96) -> (81.8, 2.96) projected
  line L315 (81.8, 2.96) -> (81.8, 105.01) projected
  line L316 (81.8, 105.01) -> (89.9, 105.01) projected
  line L317 (89.9, 105.01) -> (98.7, 105.01) projected
  line L318 (198.7, 105.01) -> (200, 105.01) projected
  line L319 (181.8, 105.01) -> (189.9, 105.01) projected
  line L320 (181.8, 2.96) -> (181.8, 105.01) projected
  line L321 (180, 2.96) -> (181.8, 2.96) projected
  line L322 (180, 105.01) -> (180, 2.96) projected
  line L323 (173.7, 105.01) -> (180, 105.01) projected
  line L324 (156.8, 105.01) -> (164.9, 105.01) projected
  line L325 (156.8, 2.96) -> (156.8, 105.01) projected
  line L326 (155, 2.96) -> (156.8, 2.96) projected
  line L327 (155, 105.01) -> (155, 2.96) projected
  line L328 (148.7, 105.01) -> (155, 105.01) projected
  line L329 (131.8, 105.01) -> (139.9, 105.01) projected
  line L330 (131.8, 2.96) -> (131.8, 105.01) projected
  line L331 (130, 2.96) -> (131.8, 2.96) projected
  line L332 (130, 105.01) -> (130, 2.96) projected
  line L333 (123.7, 105.01) -> (130, 105.01) projected
  line L334 (106.8, 105.01) -> (114.9, 105.01) projected
  line L335 (106.8, 2.96) -> (106.8, 105.01) projected
  line L336 (105, 2.96) -> (106.8, 2.96) projected
  line L337 (105, 105.01) -> (105, 2.96) projected
  line L338 (98.7, 105.01) -> (105, 105.01) projected
  line L339 (14.9, 105.01) -> (23.7, 105.01) projected
  line L340 (39.9, 105.01) -> (48.7, 105.01) projected
  line L341 (64.9, 105.01) -> (73.7, 105.01) projected
  line L342 (189.9, 105.01) -> (198.7, 105.01) projected
  line L343 (164.9, 105.01) -> (173.7, 105.01) projected
  line L344 (139.9, 105.01) -> (148.7, 105.01) projected
  line L345 (114.9, 105.01) -> (123.7, 105.01) projected
  line L346 (200, 106.61) -> (210, 106.61) projected
  line L347 (210, 106.61) -> (210, -8.64) projected
  line L348 (210, -8.64) -> (-10, -8.64) projected
  line L349 (-10, -8.64) -> (-10, 106.61) projected
  line L350 (-10, 106.61) -> (0, 106.61) projected
  line L351 (200, 105.01) -> (200, 106.61) projected
  line L352 (6.8, 2.96) -> (6.8, 105.01) projected
  line L353 (6.8, 105.01) -> (14.9, 105.01) projected
  line L354 (23.7, 105.01) -> (30, 105.01) projected
  line L355 (30, 105.01) -> (30, 2.96) projected
  line L356 (30, 2.96) -> (31.8, 2.96) projected
  line L357 (31.8, 2.96) -> (31.8, 105.01) projected
  line L358 (31.8, 105.01) -> (39.9, 105.01) projected
  line L359 (48.7, 105.01) -> (55, 105.01) projected
  line L360 (55, 105.01) -> (55, 2.96) projected
  line L361 (55, 2.96) -> (56.8, 2.96) projected
  line L362 (56.8, 2.96) -> (56.8, 105.01) projected
  line L363 (56.8, 105.01) -> (64.9, 105.01) projected
  line L364 (73.7, 105.01) -> (80, 105.01) projected
  line L365 (80, 105.01) -> (80, 2.96) projected
  line L366 (80, 2.96) -> (81.8, 2.96) projected
  line L367 (81.8, 2.96) -> (81.8, 105.01) projected
  line L368 (81.8, 105.01) -> (89.9, 105.01) projected
  line L369 (89.9, 105.01) -> (98.7, 105.01) projected
  line L370 (198.7, 105.01) -> (200, 105.01) projected
  line L371 (181.8, 105.01) -> (189.9, 105.01) projected
  line L372 (181.8, 2.96) -> (181.8, 105.01) projected
  line L373 (180, 2.96) -> (181.8, 2.96) projected
  line L374 (180, 105.01) -> (180, 2.96) projected
  line L375 (173.7, 105.01) -> (180, 105.01) projected
  line L376 (156.8, 105.01) -> (164.9, 105.01) projected
  line L377 (156.8, 2.96) -> (156.8, 105.01) projected
  line L378 (155, 2.96) -> (156.8, 2.96) projected
  line L379 (155, 105.01) -> (155, 2.96) projected
  line L380 (148.7, 105.01) -> (155, 105.01) projected
  line L381 (131.8, 105.01) -> (139.9, 105.01) projected
  line L382 (131.8, 2.96) -> (131.8, 105.01) projected
  line L383 (130, 2.96) -> (131.8, 2.96) projected
  line L384 (130, 105.01) -> (130, 2.96) projected
  line L385 (123.7, 105.01) -> (130, 105.01) projected
  line L386 (106.8, 105.01) -> (114.9, 105.01) projected
  line L387 (106.8, 2.96) -> (106.8, 105.01) projected
  line L388 (105, 2.96) -> (106.8, 2.96) projected
  line L389 (105, 105.01) -> (105, 2.96) projected
  line L390 (98.7, 105.01) -> (105, 105.01) projected
  line L391 (14.9, 105.01) -> (23.7, 105.01) projected
  line L392 (39.9, 105.01) -> (48.7, 105.01) projected
  line L393 (64.9, 105.01) -> (73.7, 105.01) projected
  line L394 (189.9, 105.01) -> (198.7, 105.01) projected
  line L395 (164.9, 105.01) -> (173.7, 105.01) projected
  line L396 (139.9, 105.01) -> (148.7, 105.01) projected
  line L397 (114.9, 105.01) -> (123.7, 105.01) projected
  line L398 (200, 106.61) -> (210, 106.61) projected
  line L399 (210, 106.61) -> (210, -8.64) projected
  line L400 (210, -8.64) -> (-10, -8.64) projected
  line L401 (-10, -8.64) -> (-10, 106.61) projected
  line L402 (-10, 106.61) -> (0, 106.61) projected
  line L403 (200, 105.01) -> (200, 106.61) projected
  line L404 (6.8, 2.96) -> (6.8, 105.01) projected
  line L405 (6.8, 105.01) -> (14.9, 105.01) projected
  line L406 (23.7, 105.01) -> (30, 105.01) projected
  line L407 (30, 105.01) -> (30, 2.96) projected
  line L408 (30, 2.96) -> (31.8, 2.96) projected
  line L409 (31.8, 2.96) -> (31.8, 105.01) projected
  line L410 (31.8, 105.01) -> (39.9, 105.01) projected
  line L411 (48.7, 105.01) -> (55, 105.01) projected
  line L412 (55, 105.01) -> (55, 2.96) projected
  line L413 (55, 2.96) -> (56.8, 2.96) projected
  line L414 (56.8, 2.96) -> (56.8, 105.01) projected
  line L415 (56.8, 105.01) -> (64.9, 105.01) projected
  line L416 (73.7, 105.01) -> (80, 105.01) projected
  line L417 (80, 105.01) -> (80, 2.96) projected
  line L418 (80, 2.96) -> (81.8, 2.96) projected
  line L419 (81.8, 2.96) -> (81.8, 105.01) projected
  line L420 (81.8, 105.01) -> (89.9, 105.01) projected
  line L421 (89.9, 105.01) -> (98.7, 105.01) projected
  line L422 (198.7, 105.01) -> (200, 105.01) projected
  line L423 (181.8, 105.01) -> (189.9, 105.01) projected
  line L424 (181.8, 2.96) -> (181.8, 105.01) projected
  line L425 (180, 2.96) -> (181.8, 2.96) projected
  line L426 (180, 105.01) -> (180, 2.96) projected
  line L427 (173.7, 105.01) -> (180, 105.01) projected
  line L428 (156.8, 105.01) -> (164.9, 105.01) projected
  line L429 (156.8, 2.96) -> (156.8, 105.01) projected
  line L430 (155, 2.96) -> (156.8, 2.96) projected
  line L431 (155, 105.01) -> (155, 2.96) projected
  line L432 (148.7, 105.01) -> (155, 105.01) projected
  line L433 (131.8, 105.01) -> (139.9, 105.01) projected
  line L434 (131.8, 2.96) -> (131.8, 105.01) projected
  line L435 (130, 2.96) -> (131.8, 2.96) projected
  line L436 (130, 105.01) -> (130, 2.96) projected
  line L437 (123.7, 105.01) -> (130, 105.01) projected
  line L438 (106.8, 105.01) -> (114.9, 105.01) projected
  line L439 (106.8, 2.96) -> (106.8, 105.01) projected
  line L440 (105, 2.96) -> (106.8, 2.96) projected
  line L441 (105, 105.01) -> (105, 2.96) projected
  line L442 (98.7, 105.01) -> (105, 105.01) projected
  line L443 (14.9, 105.01) -> (23.7, 105.01) projected
  line L444 (39.9, 105.01) -> (48.7, 105.01) projected
  line L445 (64.9, 105.01) -> (73.7, 105.01) projected
  line L446 (189.9, 105.01) -> (198.7, 105.01) projected
  line L447 (164.9, 105.01) -> (173.7, 105.01) projected
  line L448 (139.9, 105.01) -> (148.7, 105.01) projected
  line L449 (114.9, 105.01) -> (123.7, 105.01) projected
  line L450 (200, 106.61) -> (210, 106.61) projected
  line L451 (210, 106.61) -> (210, -8.64) projected
  line L452 (210, -8.64) -> (-10, -8.64) projected
  line L453 (-10, -8.64) -> (-10, 106.61) projected
  line L454 (-10, 106.61) -> (0, 106.61) projected
  line L455 (200, 105.01) -> (200, 106.61) projected
  line L456 (6.8, 2.96) -> (6.8, 105.01) projected
  line L457 (6.8, 105.01) -> (14.9, 105.01) projected
  line L458 (23.7, 105.01) -> (30, 105.01) projected
  line L459 (30, 105.01) -> (30, 2.96) projected
  line L460 (30, 2.96) -> (31.8, 2.96) projected
  line L461 (31.8, 2.96) -> (31.8, 105.01) projected
  line L462 (31.8, 105.01) -> (39.9, 105.01) projected
  line L463 (48.7, 105.01) -> (55, 105.01) projected
  line L464 (55, 105.01) -> (55, 2.96) projected
  line L465 (55, 2.96) -> (56.8, 2.96) projected
  line L466 (56.8, 2.96) -> (56.8, 105.01) projected
  line L467 (56.8, 105.01) -> (64.9, 105.01) projected
  line L468 (73.7, 105.01) -> (80, 105.01) projected
  line L469 (80, 105.01) -> (80, 2.96) projected
  line L470 (80, 2.96) -> (81.8, 2.96) projected
  line L471 (81.8, 2.96) -> (81.8, 105.01) projected
  line L472 (81.8, 105.01) -> (89.9, 105.01) projected
  line L473 (89.9, 105.01) -> (98.7, 105.01) projected
  line L474 (198.7, 105.01) -> (200, 105.01) projected
  line L475 (181.8, 105.01) -> (189.9, 105.01) projected
  line L476 (181.8, 2.96) -> (181.8, 105.01) projected
  line L477 (180, 2.96) -> (181.8, 2.96) projected
  line L478 (180, 105.01) -> (180, 2.96) projected
  line L479 (173.7, 105.01) -> (180, 105.01) projected
  line L480 (156.8, 105.01) -> (164.9, 105.01) projected
  line L481 (156.8, 2.96) -> (156.8, 105.01) projected
  line L482 (155, 2.96) -> (156.8, 2.96) projected
  line L483 (155, 105.01) -> (155, 2.96) projected
  line L484 (148.7, 105.01) -> (155, 105.01) projected
  line L485 (131.8, 105.01) -> (139.9, 105.01) projected
  line L486 (131.8, 2.96) -> (131.8, 105.01) projected
  line L487 (130, 2.96) -> (131.8, 2.96) projected
  line L488 (130, 105.01) -> (130, 2.96) projected
  line L489 (123.7, 105.01) -> (130, 105.01) projected
  line L490 (106.8, 105.01) -> (114.9, 105.01) projected
  line L491 (106.8, 2.96) -> (106.8, 105.01) projected
  line L492 (105, 2.96) -> (106.8, 2.96) projected
  line L493 (105, 105.01) -> (105, 2.96) projected
  line L494 (98.7, 105.01) -> (105, 105.01) projected
  line L495 (14.9, 105.01) -> (23.7, 105.01) projected
  line L496 (39.9, 105.01) -> (48.7, 105.01) projected
  line L497 (64.9, 105.01) -> (73.7, 105.01) projected
  line L498 (189.9, 105.01) -> (198.7, 105.01) projected
  line L499 (164.9, 105.01) -> (173.7, 105.01) projected
  line L500 (139.9, 105.01) -> (148.7, 105.01) projected
  line L501 (114.9, 105.01) -> (123.7, 105.01) projected
  line L502 (198.7, 0) -> (200, 0) projected
  line L503 (23.7, 0) -> (39.9, 0) projected
  line L504 (173.7, 0) -> (189.9, 0) projected
  line L505 (148.7, 0) -> (164.9, 0) projected
  line L506 (123.7, 0) -> (139.9, 0) projected
  line L507 (98.7, 0) -> (114.9, 0) projected
  line L508 (73.7, 0) -> (89.9, 0) projected
  line L509 (48.7, 0) -> (64.9, 0) projected
  line L510 (198.7, 0) -> (200, 0) projected
  line L511 (23.7, 0) -> (39.9, 0) projected
  line L512 (173.7, 0) -> (189.9, 0) projected
  line L513 (148.7, 0) -> (164.9, 0) projected
  line L514 (123.7, 0) -> (139.9, 0) projected
  line L515 (98.7, 0) -> (114.9, 0) projected
  line L516 (73.7, 0) -> (89.9, 0) projected
  line L517 (48.7, 0) -> (64.9, 0) projected
  line L518 (198.7, 0) -> (200, 0) projected
  line L519 (23.7, 0) -> (39.9, 0) projected
  line L520 (173.7, 0) -> (189.9, 0) projected
  line L521 (148.7, 0) -> (164.9, 0) projected
  line L522 (123.7, 0) -> (139.9, 0) projected
  line L523 (98.7, 0) -> (114.9, 0) projected
  line L524 (73.7, 0) -> (89.9, 0) projected
  line L525 (48.7, 0) -> (64.9, 0) projected
  line L526 (198.7, 0) -> (200, 0) projected
  line L527 (23.7, 0) -> (39.9, 0) projected
  line L528 (173.7, 0) -> (189.9, 0) projected
  line L529 (148.7, 0) -> (164.9, 0) projected
  line L530 (123.7, 0) -> (139.9, 0) projected
  line L531 (98.7, 0) -> (114.9, 0) projected
  line L532 (73.7, 0) -> (89.9, 0) projected
  line L533 (48.7, 0) -> (64.9, 0) projected
  line L534 (198.7, 0) -> (200, 0) projected
  line L535 (23.7, 0) -> (39.9, 0) projected
  line L536 (173.7, 0) -> (189.9, 0) projected
  line L537 (148.7, 0) -> (164.9, 0) projected
  line L538 (123.7, 0) -> (139.9, 0) projected
  line L539 (98.7, 0) -> (114.9, 0) projected
  line L540 (73.7, 0) -> (89.9, 0) projected
  line L541 (48.7, 0) -> (64.9, 0) projected
  line L542 (198.7, 0) -> (200, 0) projected
  line L543 (23.7, 0) -> (39.9, 0) projected
  line L544 (173.7, 0) -> (189.9, 0) projected
  line L545 (148.7, 0) -> (164.9, 0) projected
  line L546 (123.7, 0) -> (139.9, 0) projected
  line L547 (98.7, 0) -> (114.9, 0) projected
  line L548 (73.7, 0) -> (89.9, 0) projected
  line L549 (48.7, 0) -> (64.9, 0) projected